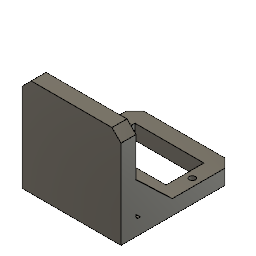
motor_mount (Autodesk Fusion 360 design; units mm, degrees)
Autodesk Fusion 360 part; units mm, degrees
note: some values were not read from the file. Set by a fixed rule: which sketch regions a step uses.
sketch "Sketch1" plane through (0, 0, 0) normal (0, 1, 0) x (1, 0, 0)
  line L0 (0, 0) -> (22.5, 0)
  line L1 (22.5, 0) -> (22.5, 12.18)
  line L2 (22.5, 12.18) -> (0, 12.18)
  line L3 (0, 12.18) -> (0, 0)
  line L4 (27.37, 0) -> (27.37, 12.18)
  line L5 (11.25, 12.18) -> (11.25, 0) construction
  line L6 (27.37, 12.18) -> (22.5, 12.18)
  line L7 (27.37, 0) -> (22.5, 0)
  circle A0 centre (25.15, 6.09) radius 1
  circle A1 centre (-2.65, 6.09) radius 1
  line L8 (-4.87, 0) -> (-4.87, 12.18)
  line L9 (-4.87, 0) -> (0, 0)
  line L10 (-4.87, 12.18) -> (0, 12.18)
  dimension "d1" = 22.5
  dimension "d3" = 4.87
  dimension "d4" = 2.65
  dimension "d11" = 2
  measures "d3" distance of L1 L4
  measures "d4" distance of L1
  measures "d11" diameter of A1
extrude "Extrude1" add sketch "Sketch1" along normal blind 15.7 contours L3 L8 L9 L10 | L1 L4 L6 L7 makes body 1 at (-4.87, 5.2333, -4.06) makes body 2 at (22.5, 5.2333, -4.06)
extrude "Extrude2" add sketch "Sketch1" along normal blind 6.7 contours A0 | A1 bodies 1 2
sketch "Sketch2" plane through (0, 15.7, 0) normal (0, 1, 0) x (-1, 0, 0)
  circle A0 centre (2.65, -6.09) radius 1
  line L0 (0, -12.18) -> (-22.5, -12.18) construction
  line L1 (-11.25, -12.18) -> (-11.25, 0) construction
  circle A1 centre (-25.15, -6.09) radius 1
  line L2 (-22.7, -12.38) -> (0.2, -12.38)
  line L3 (0.2, -12.38) -> (0.2, 0.2)
  line L4 (0.2, 0.2) -> (-22.7, 0.2)
  line L5 (-22.7, 0.2) -> (-22.7, -12.38)
  line L6 (-22.7, -12.38) -> (0.2, 0.2) construction
  line L7 (0.2, -12.38) -> (-22.7, 0.2) construction
  line L8 (-27.7, -17.38) -> (5.2, -17.38) construction
  line L9 (5.2, -17.38) -> (5.2, 5.2) construction
  line L10 (5.2, 5.2) -> (-27.7, 5.2) construction
  line L11 (-27.7, 5.2) -> (-27.7, -17.38) construction
  line L12 (-27.7, -17.38) -> (5.2, 5.2) construction
  line L13 (5.2, -17.38) -> (-27.7, 5.2) construction
  line L14 (5.2, -17.38) -> (-27.7, -17.38)
  line L15 (-27.7, -17.38) -> (-27.7, 15.2)
  line L16 (-27.7, 15.2) -> (5.2, 15.2)
  line L17 (5.2, 15.2) -> (5.2, -17.38)
  dimension "d12" = 22.9
  dimension "d13" = 12.58
  dimension "d17" = 32.9
  dimension "d18" = 22.58
  dimension "d19" = 32.58
  measures "d13" distance of origin
extrude "Extrude3" add sketch "Sketch2" along normal blind 5 separate body makes body 3
sketch "Sketch3" plane through (0, 0, 15.2) normal (0, 0, 1) x (1, 0, 0)
  line L0 (-5.2, 15.7) -> (27.7, 15.7)
  line L1 (27.7, 15.7) -> (27.7, 20.7)
  line L2 (27.7, 20.7) -> (-5.2, 20.7)
  line L3 (-5.2, 20.7) -> (-5.2, 15.7)
  line L4 (-5.2, 15.7) -> (27.7, 15.7)
  line L5 (27.7, 15.7) -> (27.7, 48.2)
  line L6 (27.7, 48.2) -> (-5.2, 48.2)
  line L7 (-5.2, 48.2) -> (-5.2, 15.7)
  dimension "d20" = 32.5
extrude "Extrude4" add sketch "Sketch3" along normal blind 5 bodies 3
sketch "Sketch4" plane through (27.7, 0, 0) normal (1, 0, 0) x (0, 0, -1)
  line L0 (-20.2, 15.7) -> (17.38, 15.7)
  line L1 (17.38, 15.7) -> (17.38, 20.7)
  line L2 (17.38, 20.7) -> (-15.2, 20.7)
  line L3 (-15.2, 20.7) -> (-15.2, 48.2)
  line L4 (-15.2, 48.2) -> (-20.2, 48.2)
  line L5 (-20.2, 48.2) -> (-20.2, 15.7)
  line L6 (17.38, 20.7) -> (-15.2, 20.7)
  line L7 (-15.2, 20.7) -> (-15.2, 48.2)
  line L8 (-20.2, 48.2) -> (-20.2, 15.7)
  line L9 (-20.2, 15.7) -> (17.38, 15.7)
  line L10 (17.38, 15.7) -> (17.38, 20.7)
  line L11 (-15.2, 48.2) -> (-20.2, 48.2)
  line L12 (-3.1667, 20.7) -> (-15.2, 32.1252)
  line L13 (-13.705, 20.7) -> (-15.2, 22.1194)
  dimension "d31" = 7.2561
  measures "d31" distance of L12 L13
sketch "Sketch5" plane through (-5.2, 0, 0) normal (-1, 0, 0) x (0, 0, 1)
  line L0 (-17.38, 15.7) -> (20.2, 15.7)
  line L1 (20.2, 15.7) -> (20.2, 48.2)
  line L2 (20.2, 48.2) -> (15.2, 48.2)
  line L3 (15.2, 48.2) -> (15.2, 20.7)
  line L4 (15.2, 20.7) -> (-17.38, 20.7)
  line L5 (-17.38, 20.7) -> (-17.38, 15.7)
  line L6 (3.1667, 20.7) -> (15.2, 32.1252)
  line L7 (13.705, 20.7) -> (15.2, 22.1194)
extrude "Extrude7" add sketch "Sketch4" against normal blind 2 contours L2 L3 L6 L7 L12 L13 bodies 3
extrude "Extrude8" add sketch "Sketch5" against normal blind 2 contours L3 L4 L6 L7 bodies 3
fillet "Fillet2" radius 0.4 4 edges at (25.7, 20.7, 8.4359) (25.7, 27.1223, 15.2) (-3.2, 27.1223, 15.2) (-3.2, 20.7, 8.4359) on bodies 3
chamfer "Chamfer1" distance 3 angle 45 4 edges at (27.7, 18.2, -17.38) (-5.2, 18.2, -17.38) (-5.2, 48.2, 17.7) (27.7, 48.2, 17.7) on bodies 3
fillet "Fillet3" radius 0.8 1 edges at (11.25, 20.7, 15.2) on bodies 3
hidden bodies 1 2
equation "d3 = ( ( 32.24 - 22.50 ) / 2 ) * 1 mm"
equation "d4 = ( ( ( 25.8 - 22.5 ) / 2 ) * 1 mm ) + 1 mm"
equation "d5 = 18.2 mm - 2.5 mm"
equation "d7 = 18.2 mm - 2.5 mm - 9 mm"
equation "d12 = 22.500 mm + 0.4 mm"
equation "d13 = 12.180 mm + 0.4 mm"
equation "d14 = thickness"
equation "thickness = 5 mm"
equation "d17 = 22.900 mm + 10 mm"
equation "d18 = 12.580 mm + 10 mm"
equation "d19 = 22.580 mm + 10 mm"
equation "d21 = thickness"
equation "d31 = 6.756108 mm + 0.5 mm"
